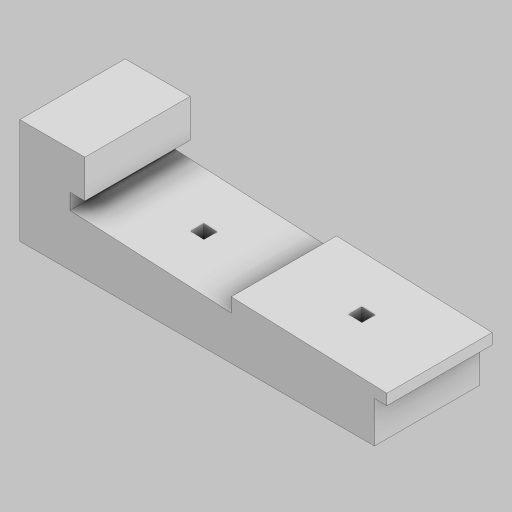
# Autodesk Inventor part: Hembra
Saved by Autodesk Inventor 2023 (Build 270158000, 158)
## iProperties
Created: 2026-02-22
Part Number: Hembra
Material: Genérico
Document SubType Name: Modeling
Designer: MARTIN MAESTRE
Density: 1 g/cm^3
Appearance: Valor por defecto
Author: MARTIN MAESTRE
Autodesk Inventor part; units mm, degrees
ref_plane "YZ Plane" through (0, 0, 0) normal (1, 0, 0) x (0, 1, 0)
ref_plane "XZ Plane" through (0, 0, 0) normal (0, 1, 0) x (-1, 0, 0)
ref_plane "XY Plane" through (0, 0, 0) normal (0, 0, 1) x (1, 0, 0)
sketch "Boceto1" plane through (0, 0, 0) normal (0, 0, 1) x (1, 0, 0)
  line L0 (0, 0) -> (134.7, 0)
  line L1 (0, 0) -> (0, 40)
  line L2 (0, 40) -> (24.7, 40)
  line L3 (24.7, 40) -> (24.7, 25.6)
  line L4 (24.7, 25.6) -> (19.1, 25.6)
  line L5 (19.1, 25.6) -> (19.1, 19.7)
  line L6 (19.1, 19.7) -> (139.4, 19.7) construction
  line L7 (134.7, 0) -> (134.7, 15.6) construction
  line L8 (134.7, 0) -> (134.7, 15.6)
  line L9 (134.7, 15.6) -> (139.4, 15.6)
  line L10 (139.4, 15.6) -> (139.4, 19.7)
  line L11 (19.1, 19.7) -> (80.3, 19.7) construction
  line L12 (80.3, 19.7) -> (80.3, 21.9) construction
  line L13 (80.3, 21.9) -> (80.3, 16.6) construction
  line L14 (19.1, 19.7) -> (80.3, 16.6)
  line L15 (80.3, 16.6) -> (80.3, 21.9)
  line L16 (80.3, 21.9) -> (139.4, 19.7)
  dimension "d0" = 134.7
  dimension "d1" = 40
  dimension "d2" = 24.7
  dimension "d3" = 14.4
  dimension "d4" = 5.6
  dimension "d5" = 5.9
  dimension "d6" = 120.3
  dimension "d7" = 15.6
  dimension "d9" = 4.7
  dimension "d10" = 61.2
  dimension "d11" = 2.2
  dimension "d12" = 5.3
  constraints: 34 end point, 5 horizontal, 4 vertical, 2 perpendicular, 2 point on line, 1 collinear
  measures "d0" distance of L0.start L0.end
  measures "d1" distance of L0.start L1.end
  measures "d2" distance of L1.end L2.end
  measures "d3" distance of L2.end L3.end
  measures "d4" distance of L3.end L4.end
  measures "d5" distance of L4.end L5.end
  measures "d6" distance of L5.end L6.end
  measures "d7" distance of L0.end L7.end
  measures "d9" distance of L7.end L9.end
  measures "d10" distance of L5.end L11.end
  measures "d11" distance of L11.end L12.end
  measures "d12" distance of L12.end L13.end
extrude "Extrusión1" add sketch "Boceto1" along normal blind 40
sketch "Boceto2" plane through (0, 0, 0) normal (0, -1, 0) x (1, 0, 0)
  line L0 (0, 0) -> (79.9, 0)
  line L1 (24.7, 0) -> (0, 0) projected
  line L2 (79.9, 0) -> (79.9, 20)
  line L3 (0, 0) -> (134.7, 0) projected
  line L4 (79.9, 0) -> (99.9, 0) construction
  line L5 (79.9, 20) -> (49.9, 20)
  line L6 (80.3, 0) -> (80.3, 40) projected
  line L7 (79.9, 20) -> (109.9, 20) construction
  line L8 (79.9, 20) -> (109.9, 20)
  line L9 (79.9, 20) -> (109.9, 20) construction
  line L10 (47.4, 17.5) -> (52.4, 17.5)
  line L11 (52.4, 17.5) -> (52.4, 22.5)
  line L12 (52.4, 22.5) -> (47.4, 22.5)
  line L13 (47.4, 22.5) -> (47.4, 17.5)
  line L14 (47.4, 17.5) -> (52.4, 22.5) construction
  line L15 (52.4, 17.5) -> (47.4, 22.5) construction
  line L16 (107.4, 17.5) -> (112.4, 17.5)
  line L17 (112.4, 17.5) -> (112.4, 22.5)
  line L18 (112.4, 22.5) -> (107.4, 22.5)
  line L19 (107.4, 22.5) -> (107.4, 17.5)
  line L20 (107.4, 17.5) -> (112.4, 22.5) construction
  line L21 (112.4, 17.5) -> (107.4, 22.5) construction
  dimension "d15" = 79.9
  dimension "d16" = 20
  dimension "d17" = 90
  dimension "d18" = 30
  dimension "d19" = 180
  dimension "d20" = 30
  dimension "d21" = 0
  dimension "d22" = 5
  dimension "d23" = 5
  dimension "d24" = 5
  dimension "d25" = 5
  constraints: 38 end point, 5 horizontal, 4 midpoint, 4 parallel, 4 perpendicular, 3 equal length, 2 collinear
  measures "d15" distance of L0.start L0.end
  measures "d16" distance of L0.end L2.end
  measures "d17" angle of L4 L2
  measures "d18" distance of L2.end L5.end
  measures "d19" angle of L5 L7
  measures "d20" distance of L2.end L7.end
  measures "d21" distance between parallel lines of L8 L9
  measures "d22" distance of L12.end L11.end
  measures "d23" distance of L11.end L10.end
  measures "d24" distance of L18.end L17.end
  measures "d25" distance of L17.end L16.end
extrude "Extrusión2" cut sketch "Boceto2" against normal blind 40 contours L13 L12 L11 L10 | L19 L18 L17 L16
